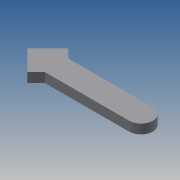
# Autodesk Inventor part: layout aide
Saved by Autodesk Inventor 2013 (Build 170138000, 138)
## iProperties
Created: 2017-03-30
Part Number: layout aide
Material: Generic
Document SubType Name: Modeling
Designer: employee
Density: 1 g/cm^3
Author: employee
Autodesk Inventor part; units mm, degrees
ref_plane "YZ Plane" through (0, 0, 0) normal (1, 0, 0) x (0, 1, 0)
ref_plane "XZ Plane" through (0, 0, 0) normal (0, 1, 0) x (-1, 0, 0)
ref_plane "XY Plane" through (0, 0, 0) normal (0, 0, 1) x (1, 0, 0)
sketch "Sketch1" plane through (0, 0, 0) normal (0, 0, 1) x (1, 0, 0)
  line L0 (0, 21.9203) -> (21.9203, 0)
  line L1 (21.9203, 0) -> (0, -21.9203)
  line L2 (0, -21.9203) -> (-21.9203, 0)
  line L3 (-21.9203, 0) -> (0, 21.9203)
  line L4 (0, 12.5) -> (99, 12.5)
  arc A0 (99, -12.5) -> (99, 12.5) centre (99, 0) ccw
  line L5 (99, -12.5) -> (0, -12.5)
  line L6 (0, -12.5) -> (0, 12.5)
  point P0 (0, 0)
  point P1 (0, 0)
  point P2 (0, 0)
  dimension "d0" = 31
  dimension "d1" = 99
  dimension "d2" = 25
  constraints: 14 end point, 2 coincident, 2 point on circle, 2 tangent, 1 centre point, 1 horizontal, 1 midpoint, 1 parallel, 1 perpendicular, 1 vertical alignment, 9 other
  measures "d0" distance between parallel lines of L1 L3
  measures "d1" distance from line of A0.centre L6
  measures "d2" distance between parallel lines of L5 L4
extrude "Extrusion1" add sketch "Sketch1" along normal blind 10
body "Solid1"
